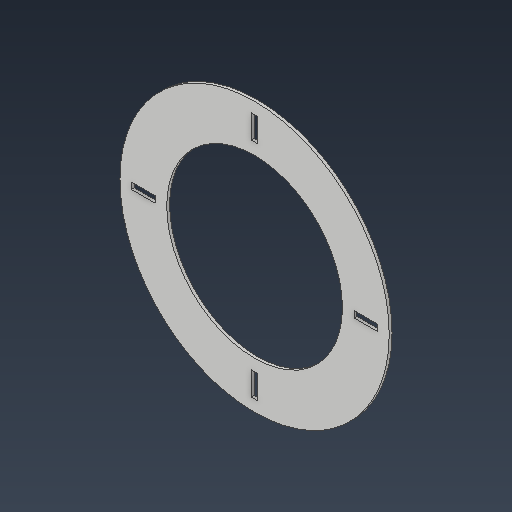
# Autodesk Inventor part: PrimaryTab
Saved by Autodesk Inventor 2021 (Build 250183000, 183)
## iProperties
Created: 2021-01-17
Part Number: PrimaryTab
Material: Типовые
Document SubType Name: Modeling
Designer: Dazer
Density: 1 g/cm^3
Appearance: По умолчанию
Author: Dazer
Autodesk Inventor part; units mm, degrees
ref_plane "YZ Plane" through (0, 0, 0) normal (1, 0, 0) x (0, 1, 0)
ref_plane "XZ Plane" through (0, 0, 0) normal (0, 1, 0) x (-1, 0, 0)
ref_plane "XY Plane" through (0, 0, 0) normal (0, 0, 1) x (1, 0, 0)
sketch "Эскиз3" plane through (0, 0, 0) normal (0, 0, 1) x (1, 0, 0)
  circle A0 centre (-46, 1.5) radius 4 projected
  circle A1 centre (-46, 1.5) radius 38 projected
  line L0 (0, 0) -> (6.5, 0) projected
  line L1 (0, 3) -> (6.5, 3) projected
  line L2 (0, 0) -> (0, 3) projected
  circle A2 centre (-46, 1.5) radius 70.8
  circle A3 centre (-46, 1.5) radius 46.2
  line L3 (6.5, 0) -> (6.5, 3) projected
  constraints: 2 centre point, 2 coincident
extrude "Выдавливание2" add sketch "Эскиз3" along normal blind 1.5 contours A3 L1 L3 L0 | A2
sketch "Эскиз4" plane through (-46, 1.5, 1.5) normal (0, 0, 1) x (1, 0, 0)
  line L0 (-46, 0) -> (-71, 0)
  line L1 (0, -46) -> (0, -71)
  line L2 (71, 0) -> (46, 0)
  line L3 (0, 52.5) -> (1.5, 52.5)
  line L4 (1.5, 52.5) -> (1.5, 64.5)
  line L5 (1.5, 64.5) -> (-1.5, 64.5)
  line L6 (-1.5, 64.5) -> (-1.5, 52.5)
  line L7 (-1.5, 52.5) -> (0, 52.5)
  line L8 (1.7, 64.7) -> (1.7, 52.3)
  line L9 (1.7, 52.3) -> (0, 52.3)
  line L10 (0, 52.3) -> (-1.7, 52.3)
  line L11 (-1.7, 52.3) -> (-1.7, 64.7)
  line L12 (-1.7, 64.7) -> (1.7, 64.7)
  line L13 (-52.3, 1.7) -> (-52.3, 0)
  line L14 (-52.5, 0) -> (-52.5, 1.5)
  line L15 (-52.3, 0) -> (-52.3, -1.7)
  line L16 (-52.5, -1.5) -> (-52.5, 0)
  line L17 (-52.5, 1.5) -> (-64.5, 1.5)
  line L18 (-64.7, 1.7) -> (-52.3, 1.7)
  line L19 (-64.5, -1.5) -> (-52.5, -1.5)
  line L20 (-52.3, -1.7) -> (-64.7, -1.7)
  line L21 (-64.7, -1.7) -> (-64.7, 1.7)
  line L22 (-64.5, 1.5) -> (-64.5, -1.5)
  line L23 (-1.7, -52.3) -> (0, -52.3)
  line L24 (0, -52.5) -> (-1.5, -52.5)
  line L25 (0, -52.3) -> (1.7, -52.3)
  line L26 (1.5, -52.5) -> (0, -52.5)
  line L27 (-1.5, -52.5) -> (-1.5, -64.5)
  line L28 (-1.7, -64.7) -> (-1.7, -52.3)
  line L29 (1.5, -64.5) -> (1.5, -52.5)
  line L30 (1.7, -52.3) -> (1.7, -64.7)
  line L31 (1.7, -64.7) -> (-1.7, -64.7)
  line L32 (-1.5, -64.5) -> (1.5, -64.5)
  line L33 (52.3, -1.7) -> (52.3, 0)
  line L34 (52.5, 0) -> (52.5, -1.5)
  line L35 (52.3, 0) -> (52.3, 1.7)
  line L36 (52.5, 1.5) -> (52.5, 0)
  line L37 (52.5, -1.5) -> (64.5, -1.5)
  line L38 (64.7, -1.7) -> (52.3, -1.7)
  line L39 (64.5, 1.5) -> (52.5, 1.5)
  line L40 (52.3, 1.7) -> (64.7, 1.7)
  line L41 (64.7, 1.7) -> (64.7, -1.7)
  line L42 (64.5, -1.5) -> (64.5, 1.5)
  point P0 (0, 0)
  dimension "d13" = 360
  constraints: 86 end point, 4 point on line, 2 perpendicular, 85 other
extrude "Выдавливание3" cut sketch "Эскиз4" against normal through all contours L15 L20 L21 L0 L22 L19 L16 | L0 L14 L17 L22 L21 L18 L13 | L16 L19 L22 L0 | L0 L22 L17 L14 | L25 L30 L31 L1 L32 L29 L26 | L1 L24 L27 L32 L31 L28 L23 | L26 L29 L32 L1 | L1 L32 L27 L24 | L34 L37 L42 L2 L41 L38 L33 | L36 L39 L42 L2 | L2 L42 L37 L34 | L2 L35 L40 L41 L42 L39 L36 | L7 L6 L5 L4 L3 | L8 L9 L10 L11 L12
